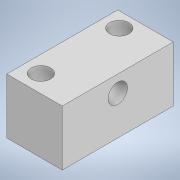
# Autodesk Inventor part: xbeltpress1
Saved by Autodesk Inventor 2020.2 (Build 242310000, 310)
## iProperties
Created: 2020-08-09
Part Number: xbeltpress1
Material: Generic
Document SubType Name: Modeling
Designer: JK
Density: 1 g/cm^3
Appearance: Default
Author: JK
Autodesk Inventor part; units mm, degrees
ref_plane "YZ Plane" through (0, 0, 0) normal (1, 0, 0) x (0, 1, 0)
ref_plane "XZ Plane" through (0, 0, 0) normal (0, 1, 0) x (-1, 0, 0)
ref_plane "XY Plane" through (0, 0, 0) normal (0, 0, 1) x (1, 0, 0)
sketch "Sketch1" plane through (0, 0, 0) normal (0, 1, 0) x (-1, 0, 0)
  line L0 (-5, 10) -> (5, 10)
  line L1 (5, 10) -> (5, -10)
  line L2 (5, -10) -> (-5, -10)
  line L3 (-5, -10) -> (-5, 10)
  line L4 (-5, 10) -> (5, -10) construction
  line L5 (5, 10) -> (-5, -10) construction
  circle A0 centre (2, 6.8502) radius 1.75
  circle A1 centre (2, -7.2838) radius 1.75
  point P0 (0, 0)
  dimension "d0" = 3.5
  dimension "d1" = 20
  dimension "d2" = 10
  dimension "d3" = 3
  constraints: 12 end point, 2 centre point, 2 midpoint, 2 parallel, 1 equal radius, 1 horizontal, 1 perpendicular, 1 vertical alignment
  measures "d0" diameter of A0
  measures "d1" distance of L0.end L1.end
  measures "d2" distance of L1.end L2.end
  measures "d3" distance from line of L1 A0.centre
extrude "Extrusion1" add sketch "Sketch1" along normal blind 10
sketch "Sketch2" plane through (5, 0, 10) normal (1, 0, 0) x (0, 0, -1)
  circle A0 centre (10, 7) radius 1.75
  line L0 (0, 10) -> (20, 10) projected
  point P0 (10, 0)
  dimension "d6" = 3.5
  dimension "d7" = 3
  constraints: 1 centre point
  measures "d6" diameter of A0
  measures "d7" distance from line of L0 A0.centre
extrude "Extrusion2" cut sketch "Sketch2" against normal blind 10
body "Solid1"
